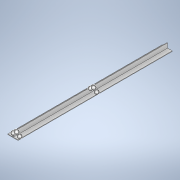
# Autodesk Inventor part: mid90
Saved by Autodesk Inventor 2020.2 (Build 242310000, 310)
## iProperties
Created: 2020-04-20
Part Number: mid90
Material: Generic
Document SubType Name: Modeling
Designer: Adam Nagy
Density: 1 g/cm^3
Appearance: Default
Author: Adam Nagy
Autodesk Inventor part; units mm, degrees
ref_plane "YZ Plane" through (0, 0, 0) normal (1, 0, 0) x (0, 1, 0)
ref_plane "XZ Plane" through (0, 0, 0) normal (0, 1, 0) x (-1, 0, 0)
ref_plane "XY Plane" through (0, 0, 0) normal (0, 0, 1) x (1, 0, 0)
sketch "Sketch1" plane through (0, 0, 0) normal (0, 0, 1) x (1, 0, 0)
  line L0 (0, 0) -> (30, 0)
  line L1 (30, 0) -> (30, 3)
  line L2 (30, 3) -> (3, 3)
  line L3 (3, 3) -> (3, 30)
  line L4 (3, 30) -> (0, 30)
  line L5 (0, 0) -> (-30, 0)
  line L6 (-30, 0) -> (-30, 3)
  line L7 (-30, 3) -> (0, 3)
  line L8 (0, 3) -> (0, 30)
  dimension "d0" = 3
  dimension "d2" = 30
  dimension "d5" = 3
  constraints: 18 end point, 6 perpendicular, 2 horizontal, 1 vertical
  measures "d0" distance between parallel lines of L0 L2
  measures "d2" distance between parallel lines of L0 L4
  measures "d5" distance between parallel lines of L5 L7
extrude "Extrusion1" add sketch "Sketch1" along normal blind 900
sketch "Sketch2" plane through (3, 3, 900) normal (0, 1, 0) x (1, 0, 0)
  line L0 (-3, 0) -> (-33, 0) projected
  line L1 (-3, 900) -> (-3, 0) projected
  line L2 (0, 900) -> (0, 0) projected
  line L3 (27, 0) -> (0, 0) projected
  point P0 (15, 15)
  point P1 (-18, 15)
  point P2 (-18, 465)
  point P3 (15, 465)
  point P4 (15, 915)
  point P5 (-18, 915)
  point P6 (-18, 1365)
  point P7 (15, 1365)
  dimension "d8" = 15
  dimension "d9" = 15
  dimension "d10" = 15
  dimension "d11" = 15
  dimension "d12" = 450
  dimension "d13" = 450
  dimension "d14" = 15
  dimension "d15" = 15
  dimension "d16" = 450
  dimension "d17" = 450
  dimension "d18" = 15
  dimension "d19" = 15
  dimension "d20" = 450
  dimension "d21" = 450
  dimension "d22" = 15
  dimension "d23" = 15
  measures "d8" distance from line of point (-18, 15) L0
  measures "d9" distance from line of point (-18, 15) L1
  measures "d10" distance from line of L2 point (15, 15)
  measures "d11" distance from line of L3 point (15, 15)
  measures "d12" distance of point (15, 465) point (15, 15)
  measures "d13" distance of point (-18, 15) point (-18, 465)
  measures "d14" distance from line of L1 point (-18, 465)
  measures "d15" distance from line of L2 point (15, 465)
  measures "d16" distance of point (15, 915) point (15, 465)
  measures "d17" distance of point (-18, 465) point (-18, 915)
  measures "d18" distance from line of L1 point (-18, 915)
  measures "d19" distance from line of L2 point (15, 915)
  measures "d20" distance of point (15, 1365) point (15, 915)
  measures "d21" distance of point (-18, 1365) point (-18, 915)
  measures "d22" distance from line of L1 point (-18, 1365)
  measures "d23" distance from line of L2 point (15, 1365)
hole "Hole1" at (18, 3, 885) at (-15, 3, 885) at (-15, 3, 435) at (18, 3, 435) at (18, 3, -15) at (-15, 3, -15) at (-15, 3, -465) at (18, 3, -465) direction (0, -1, 0) diameter 3.81 end through all
sketch "Sketch3" plane through (3, 30, 900) normal (1, 0, 0) x (0, 0, -1)
  line L0 (0, -27) -> (0, 0) projected
  line L1 (900, -27) -> (0, -27) projected
  point P0 (900, -30)
  point P1 (15, -12)
  point P2 (465, -12)
  point P3 (915, -12)
  point P4 (1365, -12)
  dimension "d31" = 15
  dimension "d32" = 15
  dimension "d33" = 450
  dimension "d34" = 15
  dimension "d35" = 450
  dimension "d36" = 450
  dimension "d37" = 15
  dimension "d38" = 15
  measures "d31" distance from line of L0 point (15, -12)
  measures "d32" distance from line of L1 point (15, -12)
  measures "d33" distance of point (465, -12) point (15, -12)
  measures "d34" distance from line of L1 point (465, -12)
  measures "d35" distance of point (465, -12) point (915, -12)
  measures "d36" distance of point (1365, -12) point (915, -12)
  measures "d37" distance from line of L1 point (915, -12)
  measures "d38" distance from line of L1 point (1365, -12)
hole "Hole2" at (3, 18, 885) at (3, 18, 435) at (3, 18, -15) at (3, 18, -465) direction (-1, 0, 0) diameter 3.81 end through all
equation "\"d0\" = Thickness"
equation "\"d2\" = Width"
equation "\"d5\" = Thickness"
equation "\"d6\" = Height"
equation "\"d8\" = HoleDistance"
equation "\"d9\" = HoleDistance"
equation "\"d10\" = HoleDistance"
equation "\"d11\" = HoleDistance"
equation "\"d14\" = HoleDistance"
equation "\"d15\" = HoleDistance"
equation "\"d18\" = HoleDistance"
equation "\"d19\" = HoleDistance"
equation "\"d22\" = HoleDistance"
equation "\"d23\" = HoleDistance"
equation "\"d31\" = HoleDistance"
equation "\"d32\" = HoleDistance"
equation "\"d34\" = HoleDistance"
equation "\"d37\" = HoleDistance"
equation "\"d38\" = HoleDistance"
equation "\"Width\" = 30"
equation "\"Thickness\" = 3"
equation "\"Height\" = 900"
equation "\"HoleDistance\" = 15"
body "Solid1"
